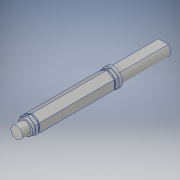
# Autodesk Inventor part: Axle1_2019
Saved by Autodesk Inventor 2019.4 (Build 234330000, 330)
## iProperties
Created: 2020-02-07
Part Number: Axle1_2019
Material: Aluminum 6061
Document SubType Name: Modeling
Designer: Paul Lefeuvre
Density: 2.7 g/cm^3
Appearance: Aluminum - Flat
Author: Paul Lefeuvre
Autodesk Inventor part; units mm, degrees
ref_plane "YZ Plane" through (0, 0, 0) normal (1, 0, 0) x (0, 1, 0)
ref_plane "XZ Plane" through (0, 0, 0) normal (0, 1, 0) x (-1, 0, 0)
ref_plane "XY Plane" through (0, 0, 0) normal (0, 0, 1) x (1, 0, 0)
sketch "Sketch1" plane through (0, 0, 0) normal (1, 0, 0) x (0, 1, 0)
  line L0 (0, 0) -> (0, -111.3)
  line L1 (4.4, 0) -> (4.4, -6.5)
  line L2 (4.4, 0) -> (0, 0)
  line L3 (5.6, -8.5) -> (6.75, -8.5)
  line L4 (6.75, -8.5) -> (6.75, -10.5)
  line L5 (6.75, -10.5) -> (5.5, -10.5)
  line L6 (5.5, -10.5) -> (5.5, -11.7)
  line L7 (5.5, -11.7) -> (6.75, -11.7)
  line L8 (6.75, -11.7) -> (6.75, -68.1)
  line L9 (6.75, -68.1) -> (5.5, -68.1)
  line L10 (5.5, -68.1) -> (5.5, -69.3)
  line L11 (5.5, -69.3) -> (6.75, -69.3)
  line L12 (6.75, -69.3) -> (6.75, -71.3)
  line L13 (6.75, -71.3) -> (7, -71.3)
  line L14 (7, -71.3) -> (7, -73.3)
  line L15 (4.4, -6.5) -> (5.6, -6.5)
  line L16 (5.6, -6.5) -> (5.6, -8.5)
  line L17 (7, -73.3) -> (5.5, -73.3)
  line L18 (5.5, -73.3) -> (5.5, -111.3)
  line L19 (5.5, -111.3) -> (0, -111.3)
  line L20 (5.5, -73.3) -> (4.5, -73.3)
  line L21 (4.5, -73.3) -> (4.5, -111.3)
  dimension "d2" = 4.4
  dimension "d3" = 2
  dimension "d4" = 1.2
  dimension "d6" = 1.2
  dimension "d7" = 2
  dimension "d8" = 5.5
  dimension "d9" = 6.75
  dimension "d10" = 6.75
  dimension "d12" = 2
  dimension "d13" = 5.5
  dimension "d14" = 5.5
  dimension "d15" = 1.5
  dimension "d16" = 6.5
  dimension "d17" = 56.4
  dimension "d18" = 2
  dimension "d19" = 38
  dimension "d20" = 1
  dimension "d24" = 5.6
  constraints: 46 end point, 13 perpendicular, 6 horizontal, 3 point on line, 2 vertical
  measures "d2" distance between parallel lines of L0 L1
  measures "d3" distance of L3.end L4.end
  measures "d4" distance of L5.end L6.end
  measures "d6" distance of L9.end L10.end
  measures "d7" distance of L11.end L12.end
  measures "d8" distance between parallel lines of L0 L6
  measures "d9" distance between parallel lines of L0 L8
  measures "d10" distance between parallel lines of L0 L4
  measures "d12" distance of L15.end L3.start
  measures "d13" distance between parallel lines of L0 L10
  measures "d14" distance between parallel lines of L0 L18
  measures "d15" distance between parallel lines of L14 L18
  measures "d16" distance of L1.start L1.end
  measures "d17" distance of L7.end L8.end
  measures "d18" distance of L13.end L14.end
  measures "d19" distance of L17.end L18.end
  measures "d20" distance of L17.end L20.end
  measures "d24" distance between parallel lines of L0 L16
revolve "Revolution1" add sketch "Sketch1" angle 360 about axis through (0, 0, 0) along (0, 0, -1)
sketch "Sketch2" plane through (0, 0, -11.7) normal (0, 0, 1) x (1, 0, 0)
  line L0 (-6.365, -3.6748) -> (-6.365, 3.6748) construction
  line L1 (-6.365, 3.6748) -> (0, 7.3497) construction
  line L2 (0, 7.3497) -> (6.365, 3.6748) construction
  line L3 (6.365, 3.6748) -> (6.365, -3.6748) construction
  line L4 (6.365, -3.6748) -> (0, -7.3497) construction
  line L5 (0, -7.3497) -> (-6.365, -3.6748) construction
  line L6 (0, 0) -> (0, 10.1619) construction
  line L7 (5.765, 3.3284) -> (0, 6.6568)
  line L8 (0, 6.6568) -> (-5.765, 3.3284)
  line L9 (-5.765, 3.3284) -> (-5.765, -3.3284)
  line L10 (-5.765, -3.3284) -> (0, -6.6568)
  line L11 (0, -6.6568) -> (5.765, -3.3284)
  line L12 (5.765, -3.3284) -> (5.765, 3.3284)
  circle A0 centre (0, 0) radius 6.7521
  point P0 (0, 0)
  dimension "d22" = 12.73
  dimension "d23" = 0.6
  constraints: 26 end point, 2 coincident, 1 centre point, 1 point on line, 1 vertical, 18 other
  measures "d22" distance of L3.end L0.start
  measures "d23" distance between parallel lines of L2 L7
extrude "Extrusion1" cut sketch "Sketch2" along normal up to surface (3.2 mm away)
extrude "Extrusion2" cut sketch "Sketch2" against normal up to surface (59.6 mm away)
sketch "Sketch3" plane through (0, 0, -111.3) normal (0, 0, -1) x (-1, 0, 0)
  circle A0 centre (0, 0) radius 5.5 projected
  line L0 (3.7749, 4) -> (-3.7749, 4)
  dimension "d31" = 1.5
  constraints: 2 end point, 2 point on circle, 1 horizontal
  measures "d31" distance edge to line of A0 L0
extrude "Extrusion4" cut sketch "Sketch3" against normal up to surface (38 mm away) contours L0 A0 picked at (-0.1977, 4.4893)
equation "\"d9\" = d10"
equation "\"d32\" = d14"
body "Solid1"
